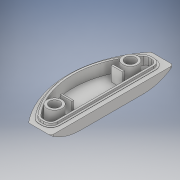
# Autodesk Inventor part: power2max_cap_v2
Saved by Autodesk Inventor 2019 (Build 230136000, 136)
## iProperties
Created: 2019-02-22
Part Number: power2max_cap_v2
Material: Generic
Document SubType Name: Modeling
Designer: jmc
Density: 1 g/cm^3
Appearance: Default
Author: jmc
Autodesk Inventor part; units mm, degrees
ref_plane "YZ Plane" through (0, 0, 0) normal (1, 0, 0) x (0, 1, 0)
ref_plane "XZ Plane" through (0, 0, 0) normal (0, 1, 0) x (-1, 0, 0)
ref_plane "XY Plane" through (0, 0, 0) normal (0, 0, 1) x (1, 0, 0)
sketch "Sketch1" plane through (0, 0, 0) normal (0, 1, 0) x (-1, 0, 0)
  line L0 (2.35, 12.1198) -> (-2.35, 12.1198)
  line L1 (2.35, -7.8802) -> (-2.35, -7.8802)
  line L2 (2.35, 12.1198) -> (2.35, 12.8198)
  line L3 (2.35, 12.8198) -> (-2.35, 12.8198)
  line L4 (-2.35, 12.8198) -> (-2.35, 12.1198)
  line L5 (2.35, -7.8802) -> (2.35, -8.5802)
  line L6 (2.35, -8.5802) -> (-2.35, -8.5802)
  line L7 (-2.35, -8.5802) -> (-2.35, -7.8802)
  circle A0 centre (0, 17.5348) radius 3.075
  circle A1 centre (0, 17.5348) radius 2.095
  line L8 (0, 12.1198) -> (0, -7.8802) construction
  line L9 (0, 2.1198) -> (9.1927, 2.1198) construction
  circle A2 centre (0, -13.2952) radius 3.075
  circle A3 centre (0, -13.2952) radius 2.095
  line L10 (0, 27.0698) -> (0, -22.8302) construction
  line L11 (8.93, 2.1198) -> (-8.93, 2.1198) construction
  line L12 (-8.01, 26.0698) -> (-8.01, -21.8302)
  line L13 (-7.01, -22.8302) -> (0.5747, -22.8302)
  line L14 (-7.01, 27.0698) -> (0.5747, 27.0698)
  arc A4 (1.2874, 26.7713) -> (0.5747, 27.0698) centre (0.5747, 26.0698) ccw
  arc A5 (-7.01, 27.0698) -> (-8.01, 26.0698) centre (-7.01, 26.0698) ccw
  arc A6 (-8.01, -21.8302) -> (-7.01, -22.8302) centre (-7.01, -21.8302) ccw
  arc A7 (0.5747, -22.8302) -> (1.2874, -22.5316) centre (0.5747, -21.8302) ccw
  line L15 (-1.3395, 23.6798) -> (-2.62, 23.6798)
  line L16 (-4.62, 21.6798) -> (-4.62, -17.4402)
  line L17 (-2.62, -19.4402) -> (-1.3395, -19.4402)
  arc A8 (0.1675, -18.755) -> (0.1675, 22.9946) centre (-23.7599, 2.1198) ccw
  arc A9 (0.1675, 22.9946) -> (-1.3395, 23.6798) centre (-1.3395, 21.6798) ccw
  arc A10 (-2.62, 23.6798) -> (-4.62, 21.6798) centre (-2.62, 21.6798) ccw
  arc A11 (-4.62, -17.4402) -> (-2.62, -19.4402) centre (-2.62, -17.4402) ccw
  arc A12 (-1.3395, -19.4402) -> (0.1675, -18.755) centre (-1.3395, -17.4402) ccw
  arc A13 (1.6746, 24.3094) -> (-1.3395, 25.6798) centre (-1.3395, 21.6798) ccw
  line L18 (-1.3395, 25.6798) -> (-2.62, 25.6798)
  arc A14 (-2.62, 25.6798) -> (-6.62, 21.6798) centre (-2.62, 21.6798) ccw
  line L19 (-6.62, 21.6798) -> (-6.62, -17.4402)
  arc A15 (-6.62, -17.4402) -> (-2.62, -21.4402) centre (-2.62, -17.4402) ccw
  line L20 (-2.62, -21.4402) -> (-1.3395, -21.4402)
  arc A16 (-1.3395, -21.4402) -> (1.6746, -20.0698) centre (-1.3395, -17.4402) ccw
  arc A17 (1.6746, -20.0698) -> (1.6746, 24.3094) centre (-23.7599, 2.1198) ccw
  arc A18 (1.2874, -22.5316) -> (1.2874, 26.7713) centre (-29.2598, 2.1198) ccw
  point P0 (0, 0)
  point P1 (0, 20.6098)
  point P2 (4.5964, 2.1198)
  point P3 (-8.01, 27.0698)
  point P4 (-8.01, -22.8302)
  point P5 (0.99, -22.8302)
  point P6 (0.99, 27.0698)
  point P7 (-0.448, 23.6798)
  point P8 (-0.448, -19.4402)
  dimension "d5" = 6.15
  dimension "d0" = 20
  dimension "d1" = 4.7
  dimension "d2" = 4.7
  dimension "d3" = 0.7
  dimension "d4" = 0.7
  dimension "d6" = 0.98
  dimension "d7" = 8.49
  dimension "d8" = 49.9
  dimension "d9" = 17.86
  dimension "d10" = 10.36
  dimension "d11" = 9
  dimension "d12" = 9
  dimension "d13" = 1
  dimension "d15" = 2
  dimension "d41" = 2
  constraints: 42 end point, 32 point on circle, 18 centre point, 14 tangent, 8 point on line, 6 equal radius, 6 horizontal, 6 midpoint, 4 perpendicular, 4 vertical, 3 coincident, 2 symmetric about line, 2 vertical alignment, 1 collinear, 1 horizontal alignment, 13 other
  measures "d0" distance between parallel lines of L1 L0
  measures "d1" distance of L1.start L1.end
  measures "d2" distance of L0.start L0.end
  measures "d3" distance of L0.start L2.end
  measures "d4" distance of L1.start L5.end
  measures "d7" distance of L8.start point (0, 20.61)
  measures "d8" distance of L10.start L10.end
  measures "d9" distance of L11.start L11.end
  measures "d10" distance from line of L12 L0.start
  measures "d11" distance of point (-8.01, -22.83) point (0.99, -22.83)
  measures "d12" distance of point (-8.01, 27.07) point (0.99, 27.07)
  measures "d13" radius of A4
  measures "d15" radius of A9
  measures "d41" radial gap between concentric circles of A8 A17
extrude "Extrusion1" add sketch "Sketch1" along normal blind 6.5 contours A0 | A2
extrude "Extrusion2" add sketch "Sketch1" along normal blind 6.27 contours L0 L4 L3 L2 | L5 L6 L7 L1
extrude "Extrusion3" add sketch "Sketch1" along normal blind 4.11 contours A17 A16 L20 A15 L19 A14 L18 A13 | A5 L14 A4 A18 A7 L13 A6 L12
sketch "Sketch2" plane through (0, 4.11, 0) normal (0, 1, 0) x (1, 0, 0)
  line L0 (4.62, 17.4402) -> (4.62, -21.6798) projected
  arc A0 (2.62, -23.6798) -> (4.62, -21.6798) centre (2.62, -21.6798) ccw projected
  line L1 (2.62, -23.6798) -> (1.3395, -23.6798) projected
  arc A1 (-0.1675, -22.9946) -> (1.3395, -23.6798) centre (1.3395, -21.6798) ccw projected
  arc A2 (-0.1675, 18.755) -> (-0.1675, -22.9946) centre (23.7599, -2.1198) ccw projected
  arc A3 (1.3395, 19.4402) -> (-0.1675, 18.755) centre (1.3395, 17.4402) ccw projected
  line L2 (1.3395, 19.4402) -> (2.62, 19.4402) projected
  arc A4 (4.62, 17.4402) -> (2.62, 19.4402) centre (2.62, 17.4402) ccw projected
  arc A5 (-0.7704, -23.5205) -> (1.3395, -24.4798) centre (1.3395, -21.6798) ccw
  line L3 (1.3395, -24.4798) -> (2.62, -24.4798)
  arc A6 (2.62, -24.4798) -> (5.42, -21.6798) centre (2.62, -21.6798) ccw
  line L4 (5.42, -21.6798) -> (5.42, 17.4402)
  arc A7 (5.42, 17.4402) -> (2.62, 20.2402) centre (2.62, 17.4402) ccw
  line L5 (2.62, 20.2402) -> (1.3395, 20.2402)
  arc A8 (1.3395, 20.2402) -> (-0.7704, 19.2809) centre (1.3395, 17.4402) ccw
  arc A9 (-0.7704, 19.2809) -> (-0.7704, -23.5205) centre (23.7599, -2.1198) ccw
  point P0 (0, 0)
  dimension "d22" = 0.8
  constraints: 10 point on circle, 6 end point, 5 centre point, 7 other
  measures "d22" radial gap between concentric circles of A2 A9
extrude "Extrusion4" add sketch "Sketch2" along normal blind 1
sketch "Sketch3" plane through (0, 4.11, 0) normal (0, 1, 0) x (1, 0, 0)
  arc A0 (-0.7704, 19.2809) -> (-0.7704, -23.5205) centre (23.7599, -2.1198) ccw projected
  arc A1 (-0.7704, -23.5205) -> (1.3395, -24.4798) centre (1.3395, -21.6798) ccw projected
  line L0 (1.3395, -24.4798) -> (2.62, -24.4798) projected
  arc A2 (2.62, -24.4798) -> (5.42, -21.6798) centre (2.62, -21.6798) ccw projected
  line L1 (5.42, -21.6798) -> (5.42, 17.4402) projected
  arc A3 (5.42, 17.4402) -> (2.62, 20.2402) centre (2.62, 17.4402) ccw projected
  line L2 (2.62, 20.2402) -> (1.3395, 20.2402) projected
  arc A4 (1.3395, 20.2402) -> (-0.7704, 19.2809) centre (1.3395, 17.4402) ccw projected
  arc A5 (-1.3732, 19.8068) -> (-1.3732, -24.0465) centre (23.7599, -2.1198) ccw
  arc A6 (1.3395, 21.0402) -> (-1.3732, 19.8068) centre (1.3395, 17.4402) ccw
  line L3 (1.3395, 21.0402) -> (2.62, 21.0402)
  arc A7 (6.22, 17.4402) -> (2.62, 21.0402) centre (2.62, 17.4402) ccw
  line L4 (6.22, 17.4402) -> (6.22, -21.6798)
  arc A8 (2.62, -25.2798) -> (6.22, -21.6798) centre (2.62, -21.6798) ccw
  line L5 (2.62, -25.2798) -> (1.3395, -25.2798)
  arc A9 (-1.3732, -24.0465) -> (1.3395, -25.2798) centre (1.3395, -21.6798) ccw
  point P0 (0, 0)
  dimension "d25" = 0.8
  constraints: 10 point on circle, 6 end point, 5 centre point, 7 other
  measures "d25" radial gap between concentric circles of A0 A5
extrude "Extrusion5" add sketch "Sketch3" along normal blind 0.1
sketch "Sketch4" plane through (0, 0, 0) normal (0, -1, 0) x (1, 0, 0)
  arc A0 (8.01, 26.0698) -> (7.01, 27.0698) centre (7.01, 26.0698) ccw projected
  line L0 (8.01, -21.8302) -> (8.01, 26.0698) projected
  line L1 (7.01, 27.0698) -> (-0.5747, 27.0698) projected
  line L2 (7.01, -22.8302) -> (-0.5747, -22.8302) projected
  arc A1 (7.01, -22.8302) -> (8.01, -21.8302) centre (7.01, -21.8302) ccw projected
  arc A2 (-0.5747, 27.0698) -> (-1.2874, 26.7713) centre (-0.5747, 26.0698) ccw projected
  arc A3 (-1.2874, -22.5316) -> (-0.5747, -22.8302) centre (-0.5747, -21.8302) ccw projected
  arc A4 (-1.2874, 26.7713) -> (-1.2874, -22.5316) centre (29.2598, 2.1198) ccw projected
  point P0 (0, 0)
extrude "Extrusion6" add sketch "Sketch4" against normal blind 0.4
sketch "Sketch5" plane through (8.01, 0, -21.8302) normal (1, 0, 0) x (0, 0, -1)
  line L0 (0, 0) -> (1, 0) construction
  line L1 (1, 0) -> (1, 4.11) construction
  line L2 (1, 4.11) -> (0, 4.11) construction
  line L3 (-47.9, 4.11) -> (0, 4.11) construction
  line L4 (-47.9, 4.11) -> (-48.9, 4.11) construction
  line L5 (-48.9, 0) -> (-48.9, 4.11) construction
  line L6 (-48.9, 0) -> (-47.9, 0) construction
  line L7 (1, 0) -> (-11, 0)
  line L8 (-48.9, 0) -> (-36.9, 0)
  arc A0 (-11, 0) -> (1, 4.11) centre (-11, 19.5732) ccw
  line L9 (1, 0) -> (1, 4.11) projected
  line L10 (1, 0) -> (1, 4.11)
  line L11 (-48.9, 0) -> (-48.9, 4.11)
  arc A1 (-48.9, 4.11) -> (-36.9, 0) centre (-36.9, 19.5732) ccw
  point P0 (-21.8302, 0)
  dimension "d30" = 12
  dimension "d31" = 12
  constraints: 8 end point, 4 point on circle, 2 centre point, 2 collinear, 2 perpendicular, 2 tangent, 1 horizontal
  measures "d30" distance of L0.end L7.end
  measures "d31" distance of L5.start L8.end
extrude "Extrusion7" cut sketch "Sketch5" against normal through all
sketch "Sketch6" plane through (8.01, 4.11, 26.0698) normal (1, 0, 0) x (0, 0, -1)
  arc A0 (36.9, -4.11) -> (47.9, -0.7266) centre (36.9, 15.4632) ccw projected
  arc A1 (0, -0.7266) -> (11, -4.11) centre (11, 15.4632) ccw projected
  arc A2 (36.9, -3.91) -> (47.7876, -0.5612) centre (36.9, 15.4632) ccw
  arc A3 (0.1124, -0.5612) -> (11, -3.91) centre (11, 15.4632) ccw
  line L0 (36.9, -4.11) -> (36.9, -3.91)
  line L1 (11, -4.11) -> (11, -3.91)
  line L2 (0.1124, -0.5612) -> (0, -0.7266)
  line L3 (47.9, -0.7266) -> (47.7876, -0.5612)
  point P0 (26.0698, -4.11)
  dimension "d37" = 0.2
  dimension "d38" = 0.2
  constraints: 8 end point, 4 point on circle, 2 centre point, 1 vertical
  measures "d37" radial gap between concentric circles of A0 A2
  measures "d38" radial gap between concentric circles of A1 A3
extrude "Extrusion8" add sketch "Sketch6" against normal through all
equation "\"d2\" = d1"
body "Solid1"
